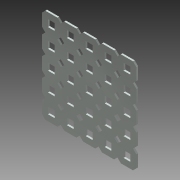
# Autodesk Inventor part: Plate 5x5 Hole
Saved by Autodesk Inventor 2013 (Build 170138000, 138)
## iProperties
Company: Autodesk Inc.
Category: Structure
Created: 2012-04-11
Document SubType Name: Sheet Metal
Designer: Autodesk Inc.
Material: Steel
Mass: 89.4134 g
Surface Area: 226.108 cm^2
Volume: 11.3902 cm^3
Density: 7.85 g/cm^3
Sheet Metal Rule: Default
Catalog Web Link: http://www.vexrobotics.com/products/accessories/structure/plate.html
Vendor: VEX
Author: Autodesk Inc.
Autodesk Inventor part; units mm, degrees
ref_plane "YZ Plane" through (0, 0, 0) normal (1, 0, 0) x (0, 1, 0)
ref_plane "XZ Plane" through (0, 0, 0) normal (0, 1, 0) x (-1, 0, 0)
ref_plane "XY Plane" through (0, 0, 0) normal (0, 0, 1) x (1, 0, 0)
sketch "Sketch1" plane through (0, 0, 0) normal (0, 0, 1) x (1, 0, 0)
  line L0 (-15.4461, 9.7381) -> (-23.5841, 9.7381)
  line L1 (-25.8651, 7.4571) -> (-25.8651, -0.6809)
  line L2 (-23.5841, -2.9619) -> (-15.4461, -2.9619)
  line L3 (-13.1651, -0.6809) -> (-13.1651, 7.4571)
  line L4 (-25.8651, 7.4571) -> (-23.5841, 9.7381)
  line L5 (-25.8651, -0.6809) -> (-23.5841, -2.9619)
  line L6 (-15.4461, -2.9619) -> (-13.1651, -0.6809)
  line L7 (-13.1651, 7.4571) -> (-15.4461, 9.7381)
  line L8 (-21.8011, 5.6741) -> (-17.2291, 5.6741)
  line L9 (-17.2291, 5.6741) -> (-17.2291, 1.1021)
  line L10 (-17.2291, 1.1021) -> (-21.8011, 1.1021)
  line L11 (-21.8011, 1.1021) -> (-21.8011, 5.6741)
  point P0 (-13.1651, 9.7381)
  point P1 (-25.8651, -2.9619)
  point P2 (-25.8651, 9.7381)
  point P3 (-13.1651, -2.9619)
  dimension "d0" = 12.7
  dimension "d1" = 12.7
  dimension "d2" = 2.281
  dimension "d3" = 2.281
  dimension "d4" = 2.281
  dimension "d5" = 2.281
  dimension "d6" = 2.281
  dimension "d7" = 2.281
  dimension "d8" = 2.281
  dimension "d9" = 2.281
  dimension "d10" = 4.572
  dimension "d11" = 4.572
  dimension "d12" = 4.064
  dimension "d13" = 4.064
  measures "d0" distance of point (-25.865, 9.738) point (-25.865, -2.962)
  measures "d1" distance of point (-13.165, 9.738) point (-25.865, 9.738)
  measures "d2" distance of L1.start point (-25.865, 9.738)
  measures "d3" distance of L0.end point (-25.865, 9.738)
  measures "d4" distance of L1.end point (-25.865, -2.962)
  measures "d5" distance of L2.start point (-25.865, -2.962)
  measures "d6" distance of L2.end point (-13.165, -2.962)
  measures "d7" distance of L3.start point (-13.165, -2.962)
  measures "d8" distance of L3.end point (-13.165, 9.738)
  measures "d9" distance of L0.start point (-13.165, 9.738)
  measures "d10" distance of L10.end L8.start
  measures "d11" distance of L9.end L10.end
  measures "d12" distance between parallel lines of L0 L8
  measures "d13" distance between parallel lines of L3 L9
extrude "Plate1" add sketch "Sketch1" along normal blind 1.1684
pattern_linear "Rectangular Pattern1" count 5 spacing 12.7 along (1, 0, 0) of "Plate1"
pattern_linear "Rectangular Pattern2" count 5 spacing 12.7 along (0, 1, 0) of "Plate1", "Rectangular Pattern1"
sketch "Sketch2" plane through (-23.5841, -2.9619, 1.1684) normal (0, 0, 1) x (1, 0, 0)
  line L0 (6.355, 59.436) -> (6.355, 54.864) projected
  line L1 (6.355, 54.864) -> (1.783, 54.864) projected
  line L2 (1.783, 54.864) -> (1.783, 59.436) projected
  line L3 (1.783, 59.436) -> (6.355, 59.436) projected
  circle A0 centre (4.069, 57.15) radius 2.286
  point P0 (23.5841, 2.9619)
  constraints: 4 tangent, 1 centre point
surface extrude "ExtrusionSrf1" sketch "Sketch2" against normal up to surface (1.1684 mm away) shown no curves A0
pattern_linear "Rectangular Pattern3" count 5 spacing 12.7 along (1, 0, 0) count 5 spacing 12.7 along (0, -1, 0) of "ExtrusionSrf1"
equation "\"d3\" = d2"
equation "\"d4\" = d2"
equation "\"d5\" = d4"
equation "\"d6\" = d2"
equation "\"d7\" = d6"
equation "\"d8\" = d2"
equation "\"d9\" = d8"
equation "\"BendRadius\" = Thickness"
equation "\"BendReliefWidth\" = Thickness"
equation "\"BendReliefDepth\" = 0.5 * Thickness"
equation "\"CornerReliefSize\" = 4 * Thickness"
equation "\"MinimumRemnant\" = 2 * Thickness"
equation "\"TransitionRadius\" = BendRadius"
equation "\"d14\" = BendRadius"
equation "\"JacobiRadiusSize\" = BendRadius"
equation "\"GapSize\" = Thickness"
equation "\"Thickness\" = 1.1684"
body "Solid1"
body "Srf1"
body "Srf2"
body "Srf3"
body "Srf4"
body "Srf5"
body "Srf16"
body "Srf17"
body "Srf18"
body "Srf19"
body "Srf20"
body "Srf31"
body "Srf32"
body "Srf33"
body "Srf34"
body "Srf35"
body "Srf46"
body "Srf47"
body "Srf48"
body "Srf49"
body "Srf50"
body "Srf61"
body "Srf62"
body "Srf63"
body "Srf64"
body "Srf65"
